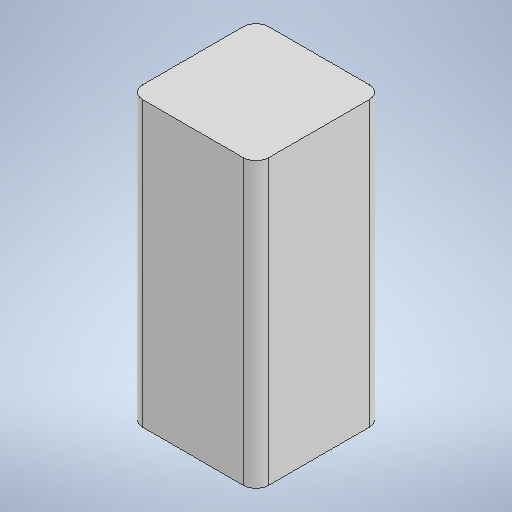
# Autodesk Inventor part: Item4040RotorVerticalV1
Saved by Autodesk Inventor 2025.1 (Build 291241000, 241)
## iProperties
Created: 2025-10-12
Part Number: Item4040RotorVerticalV1
Material: Generic
Document SubType Name: Modeling
Designer: jonas
Density: 1 g/cm^3
Appearance: Default
Author: jonas
Autodesk Inventor part; units mm, degrees
ref_plane "YZ Plane" through (0, 0, 0) normal (1, 0, 0) x (0, 1, 0)
ref_plane "XZ Plane" through (0, 0, 0) normal (0, 1, 0) x (-1, 0, 0)
ref_plane "XY Plane" through (0, 0, 0) normal (0, 0, 1) x (1, 0, 0)
sketch "Sketch1" plane through (0, 0, 0) normal (0, 1, 0) x (-1, 0, 0)
  line L0 (12.8536, 0) -> (-12.8536, 0) construction
  line L1 (0, -18.0149) -> (0, 18.0149) construction
  line L2 (16, -20) -> (-16, -20)
  line L3 (-20, -16) -> (-20, 16)
  line L4 (-16, 20) -> (16, 20)
  line L5 (20, 16) -> (20, -16)
  arc A0 (-16, 20) -> (-20, 16) centre (-16, 16) ccw
  arc A1 (-20, -16) -> (-16, -20) centre (-16, -16) ccw
  arc A2 (16, -20) -> (20, -16) centre (16, -16) ccw
  arc A3 (20, 16) -> (16, 20) centre (16, 16) ccw
  point P0 (0, 0)
  point P1 (0, 0)
  point P2 (0, 0)
  point P3 (20, -20)
  point P4 (-20, 20)
  point P5 (-20, -20)
  point P6 (20, 20)
  dimension "d0" = 40
  dimension "d1" = 40
  dimension "d2" = 4
  constraints: 12 end point, 8 point on circle, 8 point on line, 8 tangent, 4 centre point, 3 equal radius, 2 coincident, 2 horizontal, 2 midpoint, 2 parallel, 1 perpendicular, 1 vertical, 2 other
  measures "d0" distance between parallel lines of L4 L2
  measures "d1" distance between parallel lines of L5 L3
  measures "d2" radius of A0
extrude "Extrusion1" add sketch "Sketch1" along normal blind 90
body "Solid1"
